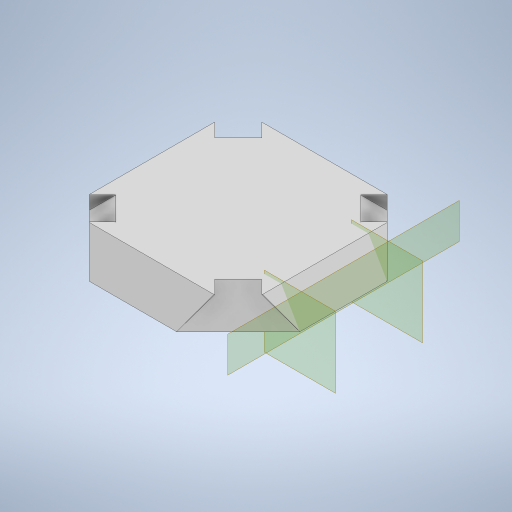
# Autodesk Inventor part: origami_linear actuator_octagon_V3(최하단) 부피구하기
Saved by Autodesk Inventor 2024 (Build 280153000, 153)
## iProperties
Created: 2023-04-11
Part Number: origami_linear actuator_octagon_V3(최하단) 부피구하기
Material: 일반
Document SubType Name: Modeling
Designer: didtk
Density: 1 g/cm^3
Appearance: 기본값
Mass: 29.8113 g
Surface Area: 87.3077 cm^2
Volume: 29.8113 cm^3
Author: didtk
Autodesk Inventor part; units mm, degrees
sketch "스케치1" plane through (0, 0, 0) normal (0, 1, 0) x (-1, 0, 0)
  line L0 (13.5, -32.5919) -> (-13.5, -32.5919)
  line L1 (-13.5, -32.5919) -> (-32.5919, -13.5)
  line L2 (-32.5919, -13.5) -> (-32.5919, 13.5)
  line L3 (-32.5919, 13.5) -> (-13.5, 32.5919)
  line L4 (-13.5, 32.5919) -> (13.5, 32.5919)
  line L5 (13.5, 32.5919) -> (32.5919, 13.5)
  line L6 (32.5919, 13.5) -> (32.5919, -13.5)
  line L7 (32.5919, -13.5) -> (13.5, -32.5919)
  point P0 (0, 0)
  point P1 (0, 0)
  point P2 (0, 32.5919)
  dimension "d0" = 27
  constraints: 16 end point, 1 coincident, 1 midpoint, 1 vertical alignment, 17 other
  measures "d0" distance of L5.end L6.end
extrude "돌출1" add sketch "스케치1" along normal blind 10
ref_plane "작업 평면1" through (13.5, 0, 32.5919) normal (0.6123724, 0.5, 0.6123724) x (0.7071068, 0, -0.7071068)
sketch "스케치2" plane through (32.5919, 0, 13.5) normal (0.7071068, 0, 0.7071068) x (0.7071068, 0, -0.7071068)
  line L0 (-27, 0) -> (0, 0) projected
  line L1 (0, 0) -> (0, 10) projected
  line L2 (-27, 10) -> (0, 10) projected
  line L3 (-27, 0) -> (-27, 10) projected
  line L4 (0, 0) -> (-8.391, 10)
  line L5 (-27, 0) -> (-18.609, 10)
  point P0 (-13.5, 0)
  dimension "d4" = 50
  dimension "d5" = 50
  constraints: 4 end point, 2 point on line
  measures "d4" angle of L0 L5
  measures "d5" angle of L0 L4
extrude "돌출2" cut sketch "스케치2" along normal up to surface contours L5 L2 L4 L0 surface through (13.5, 0, 32.5919) normal (0.6123724, 0.5, 0.6123724)
ref_plane "작업 평면2" through (32.5919, 0, 13.5) normal (0.8660254, 0.5, 0) x (0, 0, -1)
sketch "스케치3" plane through (32.5919, 0, -13.5) normal (1, 0, 0) x (0, 0, -1)
  line L0 (-27, 10) -> (0, 10) projected
  line L1 (0, 10) -> (19.0919, 10) projected
  line L2 (-32.9333, 10) -> (-27, 10) projected
  line L3 (-36.0761, 10) -> (-28.8508, 10) projected
  line L4 (-32.9333, 10) -> (-27, 0) projected
  line L5 (-27, 0) -> (-32.9333, 10)
  line L6 (-27, 0) -> (0, 0) projected
  line L7 (0, 0) -> (19.0919, 0) projected
  line L8 (0, 0) -> (5.9328, 10)
  point P0 (-13.5, 0)
  dimension "d9" = 120.682
  dimension "d10" = 120.68
  constraints: 4 end point, 1 point on line
  measures "d9" angle of L6 L4
  measures "d10" angle of L6 L8
extrude "돌출3" cut sketch "스케치3" against normal up to surface surface through (32.5919, 0, 13.5) normal (0.8660254, 0.5, 0)
ref_plane "작업 평면12" through (32.5919, 0, -13.5) normal (0, 0, -1) x (-1, 0, 0)
pattern_circular "원형 패턴1" count 4 over 360 about axis through (0, -10, 0) along (0, 1, 0) of "돌출2"
pattern_circular "원형 패턴2" count 4 over 360 about axis through (0, -10, 0) along (0, 1, 0) of "돌출3"
ref_plane "작업 평면3" through (0, 11, 0) normal (0, 1, 0) x (1, 0, 0)
ref_plane "작업 평면11" through (32.5919, 0, 13.5) normal (-1, 0, 0) x (0, 0, -1)
ref_plane "작업 평면13" through (32.5919, 0, 13.5) normal (0, 0, -1) x (-1, 0, 0)
